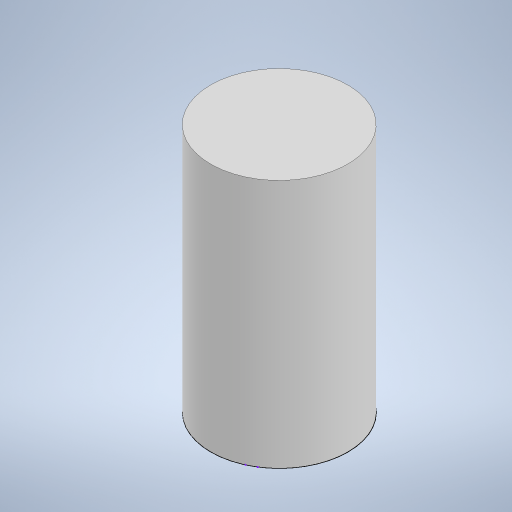
# Autodesk Inventor part: Small Peg Part
Saved by Autodesk Inventor 2023.1 (Build 271208000, 208)
## iProperties
Created: 2022-09-22
Part Number: Small Peg Part
Material: Generic
Document SubType Name: Modeling
Designer: petro
Density: 1 g/cm^3
Appearance: Default
Author: petro
Autodesk Inventor part; units mm, degrees
ref_plane "YZ Plane" through (0, 0, 0) normal (1, 0, 0) x (0, 1, 0)
ref_plane "XZ Plane" through (0, 0, 0) normal (0, 1, 0) x (-1, 0, 0)
ref_plane "XY Plane" through (0, 0, 0) normal (0, 0, 1) x (1, 0, 0)
sketch "Sketch1" plane through (0, 0, 0) normal (0, 1, 0) x (-1, 0, 0)
  circle A0 centre (0, 0) radius 0.825
  point P0 (0.8211, -0.08)
  point P1 (-0.3455, 0.7492)
  point P2 (-0.4394, 0.6983)
  point P3 (-0.4448, -0.6948)
  point P4 (-0.3436, -0.7501)
  point P5 (0.8212, 0.0791)
  dimension "d37" = 1.65
  constraints: 6 point on circle, 1 centre point, 1 coincident
  measures "d37" diameter of A0
extrude "Extrusion1" add sketch "Sketch1" along normal blind 3
body "Solid1"
